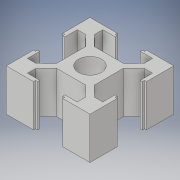
# Autodesk Inventor part: Tslot_2020extrusion_38inch
Saved by Autodesk Inventor 2018 (Build 220112000, 112)
## iProperties
Created: 2020-03-14
Part Number: Tslot_2020extrusion_38inch
Material: Generic
Document SubType Name: Modeling
Designer: natha
Density: 1 g/cm^3
Appearance: Default
Author: natha
Autodesk Inventor part; units mm, degrees
ref_plane "YZ Plane" through (0, 0, 0) normal (1, 0, 0) x (0, 1, 0)
ref_plane "XZ Plane" through (0, 0, 0) normal (0, 1, 0) x (-1, 0, 0)
ref_plane "XY Plane" through (0, 0, 0) normal (0, 0, 1) x (1, 0, 0)
sketch "Sketch1" plane through (0, 0, 0) normal (0, 1, 0) x (-1, 0, 0)
  line L0 (0, 0) -> (0, -6.5)
  line L1 (0, -6.5) -> (0.5, -6.5)
  line L2 (0.5, -6.5) -> (0.5, -7)
  line L3 (0.5, -7) -> (1, -7)
  line L4 (1, -7) -> (1, -4.05)
  line L5 (1, -4.05) -> (3, -4.05)
  line L6 (5.5, -6.5) -> (5.5, -13.5)
  line L7 (0, -13.5) -> (0.5, -13.5)
  line L8 (0.5, -13.5) -> (0.5, -13)
  line L9 (0.5, -13) -> (1, -13)
  line L10 (1, -13) -> (1, -15.95)
  line L11 (1, -15.95) -> (3, -15.95)
  line L12 (3, -15.95) -> (5.5, -13.5)
  line L13 (3, -4.05) -> (5.5, -6.5)
  line L14 (0, -13.5) -> (0, -20)
  line L15 (0, -20) -> (6.5, -20)
  line L16 (6.5, -20) -> (6.5, -19.5)
  line L17 (6.5, -19.5) -> (7, -19.5)
  line L18 (7, -19.5) -> (7, -19)
  line L19 (7, -19) -> (4.05, -19)
  line L20 (4.05, -19) -> (4.05, -17)
  line L21 (0, 0) -> (6.5, 0)
  line L22 (6.5, 0) -> (6.5, -0.5)
  line L23 (6.5, -0.5) -> (7, -0.5)
  line L24 (7, -0.5) -> (7, -1)
  line L25 (7, -1) -> (4.05, -1)
  line L26 (4.05, -1) -> (4.05, -3)
  line L27 (13.5, -20) -> (13.5, -19.5)
  line L28 (13.5, -19.5) -> (13, -19.5)
  line L29 (13, -19.5) -> (13, -19)
  line L30 (13, -19) -> (15.95, -19)
  line L31 (15.95, -19) -> (15.95, -17)
  line L32 (13.5, -14.5) -> (6.5, -14.5)
  line L33 (6.5, -14.5) -> (4.05, -17)
  line L34 (13.5, -14.5) -> (15.95, -17)
  line L35 (13.5, -20) -> (20, -20)
  line L36 (20, -20) -> (20, -13.5)
  line L37 (20, -13.5) -> (19.5, -13.5)
  line L38 (19.5, -13.5) -> (19.5, -13)
  line L39 (19.5, -13) -> (19, -13)
  line L40 (19, -13) -> (19, -15.95)
  line L41 (19, -15.95) -> (17, -15.95)
  line L42 (13.5, 0) -> (13.5, -0.5)
  line L43 (13.5, -0.5) -> (13, -0.5)
  line L44 (13, -0.5) -> (13, -1)
  line L45 (13, -1) -> (15.95, -1)
  line L46 (15.95, -1) -> (15.95, -3)
  line L47 (13.5, 0) -> (20, 0)
  line L48 (20, 0) -> (20, -6.5)
  line L49 (20, -6.5) -> (19.5, -6.5)
  line L50 (19.5, -6.5) -> (19.5, -7)
  line L51 (19.5, -7) -> (19, -7)
  line L52 (19, -7) -> (19, -4.05)
  line L53 (19, -4.05) -> (17, -4.05)
  line L54 (13.5, -5.5) -> (6.5, -5.5)
  line L55 (15.95, -3) -> (13.5, -5.5)
  line L56 (6.5, -5.5) -> (4.05, -3)
  line L57 (14.5, -6.5) -> (14.5, -13.5)
  line L58 (14.5, -13.5) -> (17, -15.95)
  line L59 (14.5, -6.5) -> (17, -4.05)
  circle A0 centre (10, -10) radius 2.75
  dimension "d0" = 6.5
  dimension "d1" = 0.5
  dimension "d2" = 0.5
  dimension "d3" = 0.5
  dimension "d4" = 2.95
  dimension "d5" = 2
  dimension "d6" = 7
  dimension "d7" = 0.5
  dimension "d8" = 2.95
  dimension "d9" = 2
  dimension "d10" = 6.5
  dimension "d11" = 6.5
  dimension "d12" = 0.5
  dimension "d13" = 0.5
  dimension "d14" = 0.5
  dimension "d15" = 2.95
  dimension "d16" = 2
  dimension "d17" = 5.5
  dimension "d18" = 6.5
  dimension "d19" = 0.5
  dimension "d20" = 0.5
  dimension "d21" = 0.5
  dimension "d22" = 2.95
  dimension "d23" = 2
  dimension "d24" = 5.5
  dimension "d25" = 0.5
  dimension "d26" = 0.5
  dimension "d27" = 0.5
  dimension "d28" = 0.5
  dimension "d29" = 2.95
  dimension "d30" = 2
  dimension "d31" = 7
  dimension "d32" = 6.5
  dimension "d33" = 6.5
  dimension "d34" = 0.5
  dimension "d35" = 0.5
  dimension "d36" = 0.5
  dimension "d37" = 2.95
  dimension "d38" = 2
  dimension "d39" = 5.5
  dimension "d40" = 5.5
  dimension "d41" = 0.5
  dimension "d42" = 0.5
  dimension "d43" = 0.5
  dimension "d44" = 2.95
  dimension "d45" = 2
  dimension "d46" = 6.5
  dimension "d47" = 6.5
  dimension "d48" = 0.5
  dimension "d49" = 0.5
  dimension "d50" = 0.5
  dimension "d51" = 2.95
  dimension "d52" = 2
  dimension "d53" = 7
  dimension "d54" = 5.5
  dimension "d55" = 5.5
  dimension "d56" = 5.5
  dimension "d57" = 5.5
  dimension "d58" = 10
  dimension "d59" = 10
  constraints: 120 end point, 40 perpendicular, 6 horizontal, 5 vertical, 1 centre point, 1 parallel
  measures "d0" distance of L0.start L0.end
  measures "d1" distance of L0.end L1.end
  measures "d2" distance of L1.end L2.end
  measures "d3" distance of L2.end L3.end
  measures "d4" distance of L3.end L4.end
  measures "d5" distance of L4.end L5.end
  measures "d6" distance of L6.start L6.end
  measures "d7" distance of L7.end L8.end
  measures "d8" distance of L9.end L10.end
  measures "d9" distance of L10.end L11.end
  measures "d10" distance of L7.start L14.end
  measures "d11" distance of L14.end L15.end
  measures "d12" distance of L15.end L16.end
  measures "d13" distance of L16.end L17.end
  measures "d14" distance of L17.end L18.end
  measures "d15" distance of L18.end L19.end
  measures "d16" distance of L19.end L20.end
  measures "d17" distance between parallel lines of L14 L6
  measures "d18" distance of L0.start L21.end
  measures "d19" distance of L21.end L22.end
  measures "d20" distance of L22.end L23.end
  measures "d21" distance of L23.end L24.end
  measures "d22" distance of L24.end L25.end
  measures "d23" distance of L25.end L26.end
  measures "d24" distance between parallel lines of L6 L0
  measures "d25" distance of L7.start L7.end
  measures "d26" distance of L27.start L27.end
  measures "d27" distance of L27.end L28.end
  measures "d28" distance of L28.end L29.end
  measures "d29" distance of L29.end L30.end
  measures "d30" distance of L30.end L31.end
  measures "d31" distance between parallel lines of L27 L16
  measures "d32" distance of L27.start L35.end
  measures "d33" distance of L35.end L36.end
  measures "d34" distance of L36.end L37.end
  measures "d35" distance of L37.end L38.end
  measures "d36" distance of L38.end L39.end
  measures "d37" distance of L39.end L40.end
  measures "d38" distance of L40.end L41.end
  measures "d39" distance between parallel lines of L35 L32
  measures "d40" distance between parallel lines of L15 L32
  measures "d41" distance of L42.start L42.end
  measures "d42" distance of L42.end L43.end
  measures "d43" distance of L43.end L44.end
  measures "d44" distance of L44.end L45.end
  measures "d45" distance of L45.end L46.end
  measures "d46" distance of L42.start L47.end
  measures "d47" distance of L47.end L48.end
  measures "d48" distance of L48.end L49.end
  measures "d49" distance of L49.end L50.end
  measures "d50" distance of L50.end L51.end
  measures "d51" distance of L51.end L52.end
  measures "d52" distance of L52.end L53.end
  measures "d53" distance between parallel lines of L42 L22
  measures "d54" distance between parallel lines of L54 L47
  measures "d55" distance between parallel lines of L54 L21
  measures "d56" distance between parallel lines of L57 L48
  measures "d57" diameter of A0
  measures "d58" distance from line of L0 A0.centre
  measures "d59" distance from line of L21 A0.centre
extrude "Extrusion1" add sketch "Sketch1" along normal blind 10
body "Solid1"
